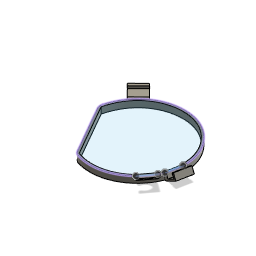
EyeTrackingLensIndex (Autodesk Fusion 360 design; units mm, degrees)
Autodesk Fusion 360 part; units mm, degrees
other "Base Mesh Feature1" in component "Original Lens Body"
sketch "Sketch1" plane through (0, 0.2, 0) normal (0, 1, 0) x (-1, 0, 0) in component "Original Lens Body"
  line L0 (10.0754, 27.2613) -> (28.7736, -5.4169)
  spline S0 degree 3 poles (28.7736, -5.4169) (28.0792, -8.2615) (26.0957, -13.8209) (20.8629, -21.008) (13.6424, -26.2058) (5.1913, -28.9419) (-3.6882, -29.1282) (-12.2204, -26.586) (-18.2549, -22.2904) (-22.2274, -17.9725) (-24.7544, -14.3669) (-26.7136, -10.42) (-27.9818, -6.1982) (-28.5541, -1.8309) (-28.4837, 4.0384) (-26.7766, 11.2487) (-22.1099, 18.8205) (-15.4149, 24.6456) (-7.3458, 28.3679) (0.0212, 29.195) (5.8518, 28.4811) (8.6812, 27.7083) (10.0754, 27.2613) knots 0 0 0 0 0.878436 1.756871 2.635307 3.513743 4.392178 5.270614 6.149049 6.588267 7.027485 7.466703 7.905921 8.345139 8.784356 9.662792 10.541228 11.419663 12.298099 13.176535 13.615752 14.05497 14.05497 14.05497 14.05497
  spline S1 degree 3 poles (29.517, -7.3073) (29.4013, -7.7765) (29.093, -8.6928) (28.4754, -10.5228) (27.5387, -12.7516) (26.2013, -15.3248) (24.6311, -17.7641) (22.8352, -20.0425) (20.1513, -22.8283) (14.7531, -26.9564) (7.3856, -29.7172) (-0.3531, -30.3011) (-6.1387, -29.65) (-11.6755, -27.8362) (-16.7331, -24.9492) (-21.1277, -21.1341) (-24.8096, -16.6335) (-27.6462, -11.5472) (-29.3301, -5.9682) (-29.886, -0.174) (-29.3763, 5.623) (-27.7804, 11.223) (-25.0959, 16.3918) (-21.4557, 20.9352) (-17.0206, 24.7032) (-11.9886, 27.6242) (-7.4076, 29.2267) (-3.6027, 29.9267) (-0.7106, 30.1609) (2.1891, 30.1043) (5.0746, 29.7831) (7.43, 29.2626) (9.3148, 28.8064) (10.5995, 28.104) (11.6216, 27.0525) (12.535, 25.3414) (15.1918, 20.7493) (19.5282, 13.2097) (24.3723, 4.8573) (27.4743, -0.6027) (28.7533, -2.9297) (29.235, -3.7685) (29.5872, -4.6703) (29.7872, -5.8776) (29.6327, -6.8381) (29.517, -7.3073) knots 0 0 0 0 0.14487 0.289741 0.579482 0.869222 1.158963 1.448704 1.738445 2.317927 3.47689 4.056372 4.635853 5.215335 5.794817 6.374298 6.95378 7.533262 8.112743 8.692225 9.271707 9.851188 10.43067 11.010152 11.589633 12.169115 12.748596 13.038337 13.328078 13.617819 13.90756 14.197301 14.342171 14.487041 14.631912 14.776782 15.066523 16.225486 17.38445 17.963931 18.108802 18.181237 18.253672 18.398543 18.543413 18.543413 18.543413 18.543413
other "MeshSection1" in component "Original Lens Body"
sketch "LensCapSketch" plane through (0, 0, 0) normal (0, 1, 0) x (1, 0, 0) in component "Lens Cap"
  spline S0 degree 3 poles (-29.517, 7.3073) (-29.4013, 7.7765) (-29.093, 8.6928) (-28.4754, 10.5228) (-27.5387, 12.7516) (-26.2013, 15.3248) (-24.6311, 17.7641) (-22.8352, 20.0425) (-20.1513, 22.8283) (-14.7531, 26.9564) (-7.3856, 29.7172) (0.3531, 30.3011) (6.1387, 29.65) (11.6755, 27.8362) (16.7331, 24.9492) (21.1277, 21.1341) (24.8096, 16.6335) (27.6462, 11.5472) (29.3301, 5.9682) (29.886, 0.174) (29.3763, -5.623) (27.7804, -11.223) (25.0959, -16.3918) (21.4557, -20.9352) (17.0206, -24.7032) (11.9886, -27.6242) (7.4076, -29.2267) (3.6027, -29.9267) (0.7106, -30.1609) (-2.1891, -30.1043) (-5.0746, -29.7831) (-7.43, -29.2626) (-9.3148, -28.8064) (-10.5995, -28.104) (-11.6216, -27.0525) (-12.535, -25.3414) (-15.1918, -20.7493) (-19.5282, -13.2097) (-24.3723, -4.8573) (-27.4743, 0.6027) (-28.7533, 2.9297) (-29.235, 3.7685) (-29.5872, 4.6703) (-29.7872, 5.8776) (-29.6327, 6.8381) (-29.517, 7.3073) knots 0 0 0 0 0.14487 0.289741 0.579482 0.869222 1.158963 1.448704 1.738445 2.317927 3.47689 4.056372 4.635853 5.215335 5.794817 6.374298 6.95378 7.533262 8.112743 8.692225 9.271707 9.851188 10.43067 11.010152 11.589633 12.169115 12.748596 13.038337 13.328078 13.617819 13.90756 14.197301 14.342171 14.487041 14.631912 14.776782 15.066523 16.225486 17.38445 17.963931 18.108802 18.181237 18.253672 18.398543 18.543413 18.543413 18.543413 18.543413
  line L0 (-10.0754, -27.2613) -> (-28.7736, 5.4169)
  spline S1 degree 3 poles (-28.7736, 5.4169) (-28.0792, 8.2615) (-26.0957, 13.8209) (-20.8629, 21.008) (-13.6424, 26.2058) (-5.1913, 28.9419) (3.6882, 29.1282) (12.2204, 26.586) (18.2549, 22.2904) (22.2274, 17.9725) (24.7544, 14.3669) (26.7136, 10.42) (27.9818, 6.1982) (28.5541, 1.8309) (28.4837, -4.0384) (26.7766, -11.2487) (22.1099, -18.8205) (15.4149, -24.6456) (7.3458, -28.3679) (-0.0212, -29.195) (-5.8518, -28.4811) (-8.6812, -27.7083) (-10.0754, -27.2613) knots 0 0 0 0 0.878436 1.756871 2.635307 3.513743 4.392178 5.270614 6.149049 6.588267 7.027485 7.466703 7.905921 8.345139 8.784356 9.662792 10.541228 11.419663 12.298099 13.176535 13.615752 14.05497 14.05497 14.05497 14.05497
  point P0 (1.264, -4.7811)
sketch "CameraHolderSketch" plane through (0, 0, 0) normal (0, 1, 0) x (1, 0, 0) in component "CameraHolder"
  line L0 (6.4443, 4.6817) -> (6.4443, -4.4768)
  line L1 (-3.5557, -4.4779) -> (-3.5557, -4.0363)
  arc A0 (-1.1335, -3.3129) -> (-1.6684, 3.0784) centre (0, 0) ccw
  spline S0 degree 3 poles (-3.5557, -4.0363) (-3.4842, -3.9822) (-3.3473, -3.8442) (-3.2224, -3.5737) (-3.0868, -3.4185) (-3.0179, -3.3424) knots 0.158022 0.158022 0.158022 0.158022 0.184788 0.215586 0.246384 0.246384 0.246384 0.246384
  arc A1 (-1.6684, 3.0784) -> (-3.1502, 3.4887) centre (-2.1464, 4.2329) cw
  line L2 (6.4443, -4.4768) -> (-3.5557, -4.4779)
  spline S1 degree 3 poles (-3.0179, -3.3424) (-2.889, -3.2319) (-2.6073, -3.036) (-2.0873, -2.9519) (-1.5961, -3.1016) (-1.2918, -3.2517) (-1.1335, -3.3129) knots 0 0 0 0 0.050913 0.101826 0.152739 0.203651 0.203651 0.203651 0.203651
  line L3 (-3.3938, 4.6817) -> (6.4443, 4.6817)
  arc A2 (-3.1502, 3.4887) -> (-3.3938, 4.6817) centre (0.6658, 4.8895) cw
  point P0 (1.2446, -4.7127)
  point P1 (6.7384, 0.924)
  point P2 (1.5, -4.5)
  point P3 (1.5, -4.5)
  dimension "d16" = 10
  constraint perpendicular L1 L2
  measures "d16" distance of L1.start L0
ref_plane "WorkPlane1" through (0.003, 4, -0.0065) normal (0, 1, 0) x (1, 0, 0) in component "EmitterHolderUpper"
extrude "Extrude1" add sketch "LensCapSketch" along normal blind 4 makes body 1 in component "Lens Cap"
sketch "LensCapBorderPlaneLine" plane through (0.003, 4, -0.0065) normal (0, 1, 0) x (1, 0, 0) in component "EmitterHolderUpper"
  line L0 (-24.5663, 17.773) -> (-17.4438, 24.7922)
  spline S0 degree 3 poles (-29.5201, 7.3008) (-29.6358, 6.8315) (-29.7903, 5.8711) (-29.5902, 4.6638) (-29.238, 3.7619) (-28.7563, 2.9232) (-27.4773, 0.5962) (-24.3754, -4.8638) (-19.5312, -13.2163) (-15.1949, -20.7559) (-12.5381, -25.3479) (-11.6247, -27.059) (-10.6026, -28.1105) (-9.3179, -28.813) (-7.433, -29.2691) (-5.0776, -29.7897) (-2.1921, -30.1109) (0.7075, -30.1675) (3.5996, -29.9332) (7.4046, -29.2333) (11.9856, -27.6307) (17.0175, -24.7098) (21.4526, -20.9418) (25.0929, -16.3983) (27.7774, -11.2295) (29.3732, -5.6295) (29.8829, 0.1675) (29.327, 5.9617) (27.6432, 11.5407) (24.8066, 16.6269) (21.1247, 21.1276) (16.73, 24.9426) (11.6725, 27.8297) (6.1356, 29.6435) (0.35, 30.2946) (-7.3886, 29.7106) (-14.7561, 26.9499) (-20.1543, 22.8217) (-22.8383, 20.0359) (-24.6342, 17.7576) (-26.2044, 15.3182) (-27.5418, 12.7451) (-28.4785, 10.5162) (-29.096, 8.6863) (-29.4044, 7.77) (-29.5201, 7.3008) knots -18.543413 -18.543413 -18.543413 -18.543413 -18.398543 -18.253672 -18.181237 -18.108802 -17.963931 -17.38445 -16.225486 -15.066523 -14.776782 -14.631912 -14.487041 -14.342171 -14.197301 -13.90756 -13.617819 -13.328078 -13.038337 -12.748596 -12.169115 -11.589633 -11.010152 -10.43067 -9.851188 -9.271707 -8.692225 -8.112743 -7.533262 -6.95378 -6.374298 -5.794817 -5.215335 -4.635853 -4.056372 -3.47689 -2.317927 -1.738445 -1.448704 -1.158963 -0.869222 -0.579482 -0.289741 -0.14487 0 0 0 0
  dimension "d26" = 10
  constraint coincident L0.start S0
  constraint coincident L0.end S0
  measures "d26" distance of L0.start L0.end
ref_plane "WorkPlane2" through (-21.002, 4, -21.2891) normal (-0.350959, -0.866025, -0.356129) x (0.712258, 0, -0.701917) in component "EmitterHolderUpper"
sketch "EmitterHolderSketchOffset" plane through (-21.002, 4, -21.2891) normal (-0.350959, -0.866025, -0.356129) x (0.712258, 0, -0.701917) in component "EmitterHolderUpper"
  line L0 (-5, 0) -> (5, 0)
  line L1 (5, 0) -> (5, -8)
  line L2 (5, -8) -> (-5, -8)
  line L3 (-5, -8) -> (-5, 0)
  line L4 (5, -6.75) -> (-5, -6.75)
  line L5 (-5, 0) -> (5, 0)
  line L6 (-5, -1.25) -> (5, -1.25)
  dimension "d32" = 1.25
  dimension "d55" = 1.25
  dimension "d66" = 10
  dimension "d67" = 8
  constraint horizontal L0
  constraint perpendicular L0 L1
  constraint perpendicular L1 L2
  constraint perpendicular L0 L3
  constraint coincident L1 L4.start
  constraint coincident L3 L4.end
  constraint perpendicular L3 L4
  constraint coincident L3 L6.start
  constraint coincident L1 L6.end
  constraint perpendicular L1 L6
  measures "d32" distance of L2 L4
  measures "d55" distance of L0 L6
  measures "d66" distance of L1.end L2.end
  measures "d67" distance of L0.start L2.end
extrude "Extrude3" add sketch "EmitterHolderSketchOffset" along normal blind 4 separate body makes body 2 in component "EmitterHolderUpper"
extrude "Extrude4" cut sketch "EmitterHolderSketchOffset" along normal blind 3 contours L1 L3 L4 L6 bodies 2 in component "EmitterHolderUpper"
revolve "Revolve1" add 1 faces at (-20.7508, 1.6906, -23.4087) angle 35 about axis through (-24.5633, 4, -17.7796) along (-0.712258, 0, 0.701917) on bodies 2 bodies 2 in component "EmitterHolderUpper"
ref_plane "WorkPlane1" through (0.003, 4, -0.0065) normal (0, 1, 0) x (1, 0, 0) in component "EmitterHolderLower"
sketch "LensCapBorderPlaneLine (2)" plane through (0.003, 4, -0.0065) normal (0, 1, 0) x (1, 0, 0) in component "EmitterHolderLower"
  line L0 (29.6932, -0.8407) -> (27.7893, -10.6578)
  spline S0 degree 3 poles (-29.5201, 7.3008) (-29.6358, 6.8315) (-29.7903, 5.8711) (-29.5902, 4.6638) (-29.238, 3.7619) (-28.7563, 2.9232) (-27.4773, 0.5962) (-24.3754, -4.8638) (-19.5312, -13.2163) (-15.1949, -20.7559) (-12.5381, -25.3479) (-11.6247, -27.059) (-10.6026, -28.1105) (-9.3179, -28.813) (-7.433, -29.2691) (-5.0776, -29.7897) (-2.1921, -30.1109) (0.7075, -30.1675) (3.5996, -29.9332) (7.4046, -29.2333) (11.9856, -27.6307) (17.0175, -24.7098) (21.4526, -20.9418) (25.0929, -16.3983) (27.7774, -11.2295) (29.3732, -5.6295) (29.8829, 0.1675) (29.327, 5.9617) (27.6432, 11.5407) (24.8066, 16.6269) (21.1247, 21.1276) (16.73, 24.9426) (11.6725, 27.8297) (6.1356, 29.6435) (0.35, 30.2946) (-7.3886, 29.7106) (-14.7561, 26.9499) (-20.1543, 22.8217) (-22.8383, 20.0359) (-24.6342, 17.7576) (-26.2044, 15.3182) (-27.5418, 12.7451) (-28.4785, 10.5162) (-29.096, 8.6863) (-29.4044, 7.77) (-29.5201, 7.3008) knots -18.543413 -18.543413 -18.543413 -18.543413 -18.398543 -18.253672 -18.181237 -18.108802 -17.963931 -17.38445 -16.225486 -15.066523 -14.776782 -14.631912 -14.487041 -14.342171 -14.197301 -13.90756 -13.617819 -13.328078 -13.038337 -12.748596 -12.169115 -11.589633 -11.010152 -10.43067 -9.851188 -9.271707 -8.692225 -8.112743 -7.533262 -6.95378 -6.374298 -5.794817 -5.215335 -4.635853 -4.056372 -3.47689 -2.317927 -1.738445 -1.448704 -1.158963 -0.869222 -0.579482 -0.289741 -0.14487 0 0 0 0
  dimension "d26_1" = 10
  constraint coincident L0.start S0
  constraint coincident L0.end S0
  measures "d26_1" distance of L0.start L0.end
ref_plane "WorkPlane2" through (28.7443, 4, 5.7427) normal (-0.490854, 0.866025, -0.095198) x (-0.190396, 0, 0.981707) in component "EmitterHolderLower"
sketch "Sketch5" plane through (28.7443, 4, 5.7427) normal (-0.490854, 0.866025, -0.095198) x (-0.190396, 0, 0.981707) in component "EmitterHolderLower"
  line L0 (-5, 0) -> (5, 0)
  line L1 (5, 0) -> (5, 8)
  line L2 (5, 8) -> (-5, 8)
  line L3 (-5, 8) -> (-5, 0)
  line L4 (-5, 6.75) -> (5, 6.75)
  line L5 (-5, 0) -> (5, 0)
  line L6 (-5, 1.25) -> (5, 1.25)
  dimension "d41" = 1.25
  dimension "d56" = 1.25
  constraint horizontal L0
  constraint vertical L1
  constraint horizontal L2
  constraint vertical L3
  constraint coincident L3 L4.start
  constraint coincident L1 L4.end
  constraint perpendicular L1 L4
  constraint coincident L3 L6.start
  constraint coincident L1 L6.end
  constraint perpendicular L1 L6
  measures "d41" distance of L2 L4
  measures "d56" distance of L0 L6
extrude "Extrude5" add sketch "Sketch5" against normal blind 4 separate body makes body 3 in component "EmitterHolderLower"
extrude "Extrude6" cut sketch "Sketch5" against normal blind 3 contours L1 L3 L4 L6 bodies 3 in component "EmitterHolderLower"
revolve "Revolve2" add 1 faces at (30.3705, 1.6906, 4.3604) angle 35 about axis through (29.6963, 4, 0.8342) along (0.190396, 0, -0.981707) on bodies 3 bodies 3 in component "EmitterHolderLower"
ref_plane "WorkPlane1" through (0.003, 4, -0.0065) normal (0, 1, 0) x (1, 0, 0) in component "CameraHolder"
sketch "AnglePlaneAxis" plane through (0.003, 4, -0.0065) normal (0, 1, 0) x (1, 0, 0) in component "CameraHolder"
  line L0 (20.4155, -21.7055) -> (26.4311, -13.7173)
  spline S0 degree 3 poles (-29.5201, 7.3008) (-29.6358, 6.8315) (-29.7903, 5.8711) (-29.5902, 4.6638) (-29.238, 3.7619) (-28.7563, 2.9232) (-27.4773, 0.5962) (-24.3754, -4.8638) (-19.5312, -13.2163) (-15.1949, -20.7559) (-12.5381, -25.3479) (-11.6247, -27.059) (-10.6026, -28.1105) (-9.3179, -28.813) (-7.433, -29.2691) (-5.0776, -29.7897) (-2.1921, -30.1109) (0.7075, -30.1675) (3.5996, -29.9332) (7.4046, -29.2333) (11.9856, -27.6307) (17.0175, -24.7098) (21.4526, -20.9418) (25.0929, -16.3983) (27.7774, -11.2295) (29.3732, -5.6295) (29.8829, 0.1675) (29.327, 5.9617) (27.6432, 11.5407) (24.8066, 16.6269) (21.1247, 21.1276) (16.73, 24.9426) (11.6725, 27.8297) (6.1356, 29.6435) (0.35, 30.2946) (-7.3886, 29.7106) (-14.7561, 26.9499) (-20.1543, 22.8217) (-22.8383, 20.0359) (-24.6342, 17.7576) (-26.2044, 15.3182) (-27.5418, 12.7451) (-28.4785, 10.5162) (-29.096, 8.6863) (-29.4044, 7.77) (-29.5201, 7.3008) knots -18.543413 -18.543413 -18.543413 -18.543413 -18.398543 -18.253672 -18.181237 -18.108802 -17.963931 -17.38445 -16.225486 -15.066523 -14.776782 -14.631912 -14.487041 -14.342171 -14.197301 -13.90756 -13.617819 -13.328078 -13.038337 -12.748596 -12.169115 -11.589633 -11.010152 -10.43067 -9.851188 -9.271707 -8.692225 -8.112743 -7.533262 -6.95378 -6.374298 -5.794817 -5.215335 -4.635853 -4.056372 -3.47689 -2.317927 -1.738445 -1.448704 -1.158963 -0.869222 -0.579482 -0.289741 -0.14487 0 0 0 0
  dimension "d49" = 10
  constraint coincident L0.end S0
  constraint coincident L0.start S0
  measures "d49" distance of L0.start L0.end
ref_plane "WorkPlane2" through (23.4264, 4, 17.7048) normal (0.513476, -0.766044, 0.386676) x (0.601562, 0, -0.798826) in component "CameraHolder"
sketch "CameraHolderOffset" plane through (23.4264, 4, 17.7048) normal (0.513476, -0.766044, 0.386676) x (0.601562, 0, -0.798826) in component "CameraHolder"
  line L0 (5, 9.1585) -> (5, 0)
  line L1 (-5, -0.0011) -> (-5.0001, 0.4405)
  spline S0 degree 3 poles (-4.4622, 1.1344) (-4.3334, 1.2449) (-4.0516, 1.4408) (-3.5316, 1.5249) (-3.0405, 1.3752) (-2.7361, 1.2251) (-2.5778, 1.1639) knots 0 0 0 0 0.050913 0.101826 0.152739 0.203651 0.203651 0.203651 0.203651
  spline S1 degree 3 poles (-5.0001, 0.4405) (-4.9285, 0.4946) (-4.7917, 0.6326) (-4.6667, 0.9031) (-4.5311, 1.0583) (-4.4622, 1.1344) knots 0.158022 0.158022 0.158022 0.158022 0.184788 0.215586 0.246384 0.246384 0.246384 0.246384
  line L2 (5, 0) -> (-5, -0.0011)
  arc A0 (-3.1127, 7.5552) -> (-4.5945, 7.9655) centre (-3.5907, 8.7097) cw
  line L3 (-4.8382, 9.1585) -> (5, 9.1585)
  arc A1 (-2.5778, 1.1639) -> (-3.1127, 7.5552) centre (-1.4443, 4.4768) ccw
  arc A2 (-4.5945, 7.9655) -> (-4.8382, 9.1585) centre (-0.7785, 9.3663) cw
  point P0 (1.2446, 4.2873)
  point P1 (6.7384, 9.924)
  point P2 (1.5, 4.5)
  point P3 (1.5, 4.5)
  point P4 (0, 9)
  point P5 (5, 0)
  dimension "d51" = 10
  constraint perpendicular L1 L2
  constraint coincident P5 L0.end
  measures "d51" distance of L1.start L0
extrude "Extrude2" add sketch "CameraHolderOffset" along normal blind 2 separate body makes body 4 in component "CameraHolder"
revolve "Revolve1'" add 1 faces at (22.7656, 3.4888, 19.2936) angle 35 about axis through (20.4186, 4, 21.699) along (0.601562, 0, -0.798826) on bodies 4 bodies 4 in component "CameraHolder"
ref_plane "WorkPlane1" through (-52, 0, 0) normal (1, 0, 0) x (0, 1, 0) in component "Left Lens Cap"
mirror "Mirror2" about plane through (-52, 0, 0) normal (1, 0, 0) of bodies 1 makes body 5 in component "Lens Cap"
mirror "Mirror2'" about plane through (-52, 0, 0) normal (1, 0, 0) of bodies 4 makes body 6 in component "CameraHolder"
mirror "Mirror2''" about plane through (-52, 0, 0) normal (1, 0, 0) of bodies 2 makes body 7 in component "EmitterHolderUpper"
mirror "Mirror2'''" about plane through (-52, 0, 0) normal (1, 0, 0) of bodies 3 makes body 8 in component "EmitterHolderLower"
component "Original Lens Body" placed x (1, 0, 0) y (0, 1, 0) z (0, 0, 1) at (0, 0, 0)
component "Lens Cap" placed x (1, 0, 0) y (0, 1, 0) z (0, 0, 1) at (0, 0, 0)
component "CameraHolder" placed x (1, 0, 0) y (0, 1, 0) z (0, 0, 1) at (0, 0, 0)
component "EmitterHolderUpper" placed x (1, 0, 0) y (0, 1, 0) z (0, 0, 1) at (0, 0, 0)
component "EmitterHolderLower" placed x (1, 0, 0) y (0, 1, 0) z (0, 0, 1) at (0, 0, 0)
component "Left Lens Cap" placed x (1, 0, 0) y (0, 1, 0) z (0, 0, 1) at (0, 0, 0)
hidden bodies 5 6 7 8
